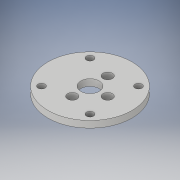
# Autodesk Inventor part: フランジ
Saved by Autodesk Inventor 2019 (Build 230136000, 136)
## iProperties
Created: 2020-10-25
Part Number: フランジ
Material: 一般
Document SubType Name: Modeling
Designer: zhept
Density: 1 g/cm^3
Appearance: 既定
Author: zhept
Autodesk Inventor part; units mm, degrees
ref_plane "YZ Plane" through (0, 0, 0) normal (1, 0, 0) x (0, 1, 0)
ref_plane "XZ Plane" through (0, 0, 0) normal (0, 1, 0) x (-1, 0, 0)
ref_plane "XY Plane" through (0, 0, 0) normal (0, 0, 1) x (1, 0, 0)
sketch "スケッチ1" plane through (0, 0, 0) normal (0, 1, 0) x (-1, 0, 0)
  circle A0 centre (0, 0) radius 19
  line L0 (0, 0) -> (0, 8)
  line L1 (0, 0) -> (-8, 0)
  line L2 (0, 0) -> (0, -8)
  circle A1 centre (0, -8) radius 2.15
  circle A2 centre (0, 8) radius 2.15
  circle A3 centre (-8, 0) radius 2.15
  dimension "d0" = 38
  dimension "d1" = 8
  dimension "d2" = 8
  dimension "d4" = 8
  dimension "d5" = 4.3
  dimension "d6" = 4.3
  dimension "d7" = 4.3
  constraints: 6 end point, 4 centre point, 4 coincident, 2 vertical, 1 horizontal
  measures "d0" diameter of A0
  measures "d1" distance of L0.start L0.end
  measures "d2" distance of L0.start L1.end
  measures "d4" distance of L0.start L2.end
  measures "d5" diameter of A1
  measures "d6" diameter of A2
  measures "d7" diameter of A3
extrude "押し出し1" add sketch "スケッチ1" along normal blind 3
sketch "スケッチ3" plane through (0, 3, 0) normal (0, 1, 0) x (1, 0, 0)
  circle A0 centre (0, 0) radius 4.15
  dimension "d24" = 8.3
  constraints: 1 centre point, 1 coincident
  measures "d24" diameter of A0
extrude "押し出し3" cut sketch "スケッチ3" against normal blind 10
sketch "スケッチ4" plane through (0, 3, 0) normal (0, 1, 0) x (1, 0, 0)
  line L0 (0, 0) -> (-10.9602, 10.9602)
  line L1 (0, 0) -> (15.5, 0) construction
  circle A0 centre (-10.9602, 10.9602) radius 1.6
  line L2 (0, 0) -> (10.9494, 10.9709)
  circle A1 centre (10.9494, 10.9709) radius 1.6
  line L3 (0, 0) -> (-10.9731, -10.9472)
  circle A2 centre (-10.9731, -10.9472) radius 1.6
  line L4 (0, 0) -> (10.9602, -10.9602)
  line L5 (0, 0) -> (15.5, 0) construction
  circle A3 centre (10.9602, -10.9602) radius 1.6
  circle A4 centre (0, 0) radius 12.5
  dimension "d27" = 15.5
  dimension "d28" = 135
  dimension "d29" = 3.2
  dimension "d30" = 15.5
  dimension "d31" = 3.2
  dimension "d32" = 15.5
  dimension "d33" = 3.2
  dimension "d34" = 15.5
  dimension "d35" = 45
  dimension "d36" = 3.2
  dimension "d37" = 25
  constraints: 12 end point, 6 coincident, 5 centre point, 2 equal length, 2 horizontal
  measures "d27" distance of L0.start L0.end
  measures "d28" angle of L1 L0
  measures "d29" diameter of A0
  measures "d30" distance of L0.start L2.end
  measures "d31" diameter of A1
  measures "d32" distance of L0.start L3.end
  measures "d33" diameter of A2
  measures "d34" distance of L0.start L4.end
  measures "d35" angle of L4 L5
  measures "d36" diameter of A3
  measures "d37" diameter of A4
extrude "押し出し4" cut sketch "スケッチ4" against normal blind 10 contours A0 | A1 | A2 | A3
